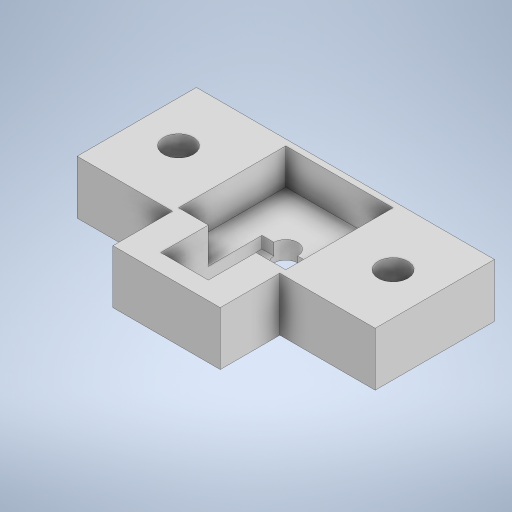
# Autodesk Inventor part: gps_holder
Saved by Autodesk Inventor 2024 (Build 280153000, 153)
## iProperties
Created: 2025-12-27
Part Number: gps_holder
Material: Generic
Document SubType Name: Modeling
Designer: schar
Density: 1 g/cm^3
Appearance: Default
Author: schar
Autodesk Inventor part; units mm, degrees
ref_plane "YZ Plane" through (0, 0, 0) normal (1, 0, 0) x (0, 1, 0)
ref_plane "XZ Plane" through (0, 0, 0) normal (0, 1, 0) x (-1, 0, 0)
ref_plane "XY Plane" through (0, 0, 0) normal (0, 0, 1) x (1, 0, 0)
sketch "Sketch1" plane through (0, 0, 0) normal (0, 1, 0) x (-1, 0, 0)
  line L0 (9, 9) -> (-9, 9)
  line L1 (-9, 9) -> (-9, -9)
  line L2 (-9, -9) -> (9, -9)
  line L3 (9, -9) -> (9, 9)
  line L4 (9, 9) -> (-9, -9) construction
  line L5 (-9, 9) -> (9, -9) construction
  line L6 (25, 10) -> (-25, 10)
  line L7 (-25, 10) -> (-25, -10)
  line L8 (-25, -10) -> (25, -10)
  line L9 (25, -10) -> (25, 10)
  line L10 (25, 10) -> (-25, -10) construction
  line L11 (-25, 10) -> (25, -10) construction
  line L12 (25, 0) -> (18, 0)
  line L13 (-25, 0) -> (-18, 0)
  circle A0 centre (18, 0) radius 2.5
  circle A1 centre (-18, 0) radius 2.5
  point P0 (0, 0)
  dimension "d0" = 18
  dimension "d1" = 18
  dimension "d2" = 50
  dimension "d3" = 20
  dimension "d4" = 7
  dimension "d5" = 5
  dimension "d6" = 5
  constraints: 28 end point, 6 midpoint, 4 horizontal, 4 parallel, 2 centre point, 2 coincident, 2 perpendicular
  measures "d0" distance of L2.end L1.end
  measures "d1" distance of L1.end L0.end
  measures "d2" distance of L8.end L7.end
  measures "d3" distance of L7.end L6.end
  measures "d4" distance of L12.start L12.end
  measures "d5" diameter of A0
  measures "d6" diameter of A1
extrude "Extrusion1" add sketch "Sketch1" along normal blind 3 contours L3 L2 L1 L0 | L9 L8 L7 L6
sketch "Sketch2" plane through (0, 3, 0) normal (0, 1, 0) x (1, 0, 0)
  line L0 (-9, 9) -> (9, 9)
  line L1 (9, 9) -> (9, -9)
  line L2 (9, -9) -> (-9, -9)
  line L3 (-9, -9) -> (-9, 9)
  line L4 (-9, 9) -> (9, -9) construction
  line L5 (9, 9) -> (-9, -9) construction
  circle A0 centre (-18, 0) radius 2.5
  circle A1 centre (18, 0) radius 2.5
  line L6 (-25, -10) -> (25, -10) projected
  line L7 (-25, 10) -> (25, 10)
  line L8 (25, 10) -> (25, -10)
  line L9 (25, -10) -> (-25, -10)
  line L10 (-25, -10) -> (-25, 10)
  line L11 (-25, 10) -> (25, -10) construction
  line L12 (25, 10) -> (-25, -10) construction
  point P0 (0, 0)
  dimension "d9" = 18
  dimension "d10" = 18
  constraints: 24 end point, 4 midpoint, 4 parallel, 2 centre point, 2 horizontal, 2 perpendicular
  measures "d9" distance of L1.end L2.end
  measures "d10" distance of L0.end L1.end
extrude "Extrusion2" add sketch "Sketch2" along normal blind 6
sketch "Sketch3" plane through (-25, 0, 10) normal (0, 0, 1) x (1, 0, 0)
  line L0 (34, 3) -> (34, 9) projected
  line L1 (16, -9) -> (34, -9)
  line L2 (34, -9) -> (34, 9)
  line L3 (34, 9) -> (16, 9)
  line L4 (16, 9) -> (16, -9)
  line L5 (16, -9) -> (34, 9) construction
  line L6 (34, -9) -> (16, 9) construction
  line L7 (16, 0) -> (34, 0)
  point P0 (25, 0)
  constraints: 14 end point, 4 midpoint, 2 parallel, 1 horizontal, 1 perpendicular
extrude "Extrusion3" add sketch "Sketch3" along normal blind 10 contours L2 L7 L4 L3 L0
sketch "Sketch4" plane through (0, 9, 0) normal (0, 1, 0) x (1, 0, 0)
  line L0 (-9, -9) -> (9, -9) projected
  line L1 (0, -9) -> (0, -13)
  line L2 (4, -17) -> (-4, -17)
  line L3 (-4, -17) -> (-4, -9)
  line L4 (-4, -9) -> (4, -9)
  line L5 (4, -9) -> (4, -17)
  line L6 (4, -17) -> (-4, -9) construction
  line L7 (-4, -17) -> (4, -9) construction
  point P0 (0, 0)
  dimension "d15" = 4
  dimension "d16" = 8
  constraints: 14 end point, 3 midpoint, 2 parallel, 1 horizontal, 1 perpendicular, 1 point on line, 1 vertical
  measures "d15" distance of L1.start L1.end
  measures "d16" distance of L3.end L4.end
extrude "Extrusion4" cut sketch "Sketch4" against normal blind 8
sketch "Sketch5" plane through (0, 3, 0) normal (0, 1, 0) x (1, 0, 0)
  line L0 (-4, -9) -> (4, -9) projected
  line L1 (0, -9) -> (0, -6)
  line L2 (0, -6) -> (-4, -6)
  line L3 (-4, -6) -> (-4, -9)
  line L4 (-4, -9) -> (0, -9)
  line L5 (0, -9) -> (0, -6)
  line L6 (0, -6) -> (4, -6)
  line L7 (4, -6) -> (4, -9)
  line L8 (4, -9) -> (0, -9)
  line L9 (0, -9) -> (0, -6)
  line L10 (-4, -6) -> (4, -6)
  line L11 (4, -6) -> (4, 0)
  line L12 (4, 0) -> (-4, 0)
  line L13 (-4, 0) -> (-4, -6)
  point P0 (0, 0)
  dimension "d19" = 3
  constraints: 26 end point, 6 parallel, 3 horizontal, 3 perpendicular, 1 midpoint, 1 vertical
  measures "d19" distance of L1.start L1.end
extrude "Extrusion5" cut sketch "Sketch5" against normal blind 2
sketch "Sketch6" plane through (0, 3, 0) normal (0, 1, 0) x (1, 0, 0)
  circle A0 centre (0, 0) radius 2
  dimension "d22" = 4
  constraints: 1 centre point, 1 coincident
  measures "d22" diameter of A0
extrude "Extrusion6" cut sketch "Sketch6" against normal through all
body "Solid1"
